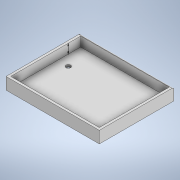
# Autodesk Inventor part: Part4
Saved by Autodesk Inventor 2022 (Build 260153000, 153)
## iProperties
Created: 2022-05-05
Part Number: Part4
Material: Generic
Document SubType Name: Modeling
Designer: Asus
Density: 1 g/cm^3
Appearance: Default
Author: Asus
Autodesk Inventor part; units mm, degrees
ref_plane "YZ Plane" through (0, 0, 0) normal (1, 0, 0) x (0, 1, 0)
ref_plane "XZ Plane" through (0, 0, 0) normal (0, 1, 0) x (-1, 0, 0)
ref_plane "XY Plane" through (0, 0, 0) normal (0, 0, 1) x (1, 0, 0)
sketch "Sketch1" plane through (0, 0, 0) normal (0, 1, 0) x (-1, 0, 0)
  line L0 (53.9548, -48.6252) -> (-46.0452, -48.6252)
  line L1 (-46.0452, -48.6252) -> (-46.0452, -128.6252)
  line L2 (-46.0452, -128.6252) -> (53.9548, -128.6252)
  line L3 (53.9548, -128.6252) -> (53.9548, -48.6252)
  point P0 (0, 0)
  dimension "d6" = 100
  dimension "d7" = 80
  constraints: 8 end point, 2 parallel, 1 horizontal, 1 perpendicular
  measures "d6" distance of L1.end L2.end
  measures "d7" distance of L2.end L0.start
extrude "Extrusion1" add sketch "Sketch1" along normal blind 12.7
shell "Shell1" thickness 2.54 removed faces 1 at (12.7119, 12.7, -75.2919)
fillet "Fillet1" radius 2 1 edges at (-3.9548, 12.7, -128.6252)
sketch "Sketch2" plane through (-51.4148, 2.54, -126.0852) normal (0, 1, 0) x (1, 0, 0)
  circle A0 centre (11.4204, -24.6498) radius 2.5
  point P0 (51.4148, -126.0852)
  dimension "d8" = 5
  constraints: 1 centre point
  measures "d8" diameter of A0
extrude "Extrusion2" cut sketch "Sketch2" against normal blind 10
body "Solid1"
